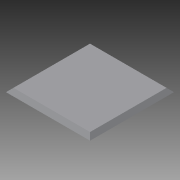
# Autodesk Inventor part: Element
Saved by Autodesk Inventor 2015 (Build 190159000, 159)
## iProperties
Created: 2016-03-23
Part Number: Element
Material: Generic
Document SubType Name: Modeling
Designer: Noah
Density: 1 g/cm^3
Appearance: Default
Author: Noah
Autodesk Inventor part; units mm, degrees
ref_plane "YZ Plane" through (0, 0, 0) normal (1, 0, 0) x (0, 1, 0)
ref_plane "XZ Plane" through (0, 0, 0) normal (0, 1, 0) x (-1, 0, 0)
ref_plane "XY Plane" through (0, 0, 0) normal (0, 0, 1) x (1, 0, 0)
sketch "Sketch1" plane through (0, 0, 0) normal (0, 0, 1) x (1, 0, 0)
  line L0 (-180, 180) -> (180, 180)
  line L1 (180, 180) -> (180, -180)
  line L2 (180, -180) -> (-180, -180)
  line L3 (-180, -180) -> (-180, 180)
  point P0 (0, 0)
  dimension "d0" = 360
  dimension "d1" = 360
  dimension "d2" = 180
  dimension "d3" = 180
  constraints: 8 end point, 2 parallel, 1 horizontal, 1 perpendicular
  measures "d0" distance of L0.start L0.end
  measures "d1" distance of L2.end L0.start
  measures "d2" distance from line of point (0, 0) L1
  measures "d3" distance from line of point (0, 0) L0
extrude "Extrusion1" add sketch "Sketch1" along normal blind 16
chamfer "Chamfer1" distance 16 angle 45 4 edges at (-180, 0, 16) (0, -180, 16) (180, 0, 16) (0, 180, 16)
equation "\"d0\" = edge_length_1"
equation "\"d1\" = edge_length_1"
equation "\"d2\" = 0.5 * edge_length_1"
equation "\"d3\" = 0.5 * edge_length_1"
equation "\"d4\" = wall_width_1"
equation "\"d6\" = wall_width_1"
equation "\"edge_length_1\" = 360"
equation "\"wall_width_1\" = 16"
body "Solid1"
